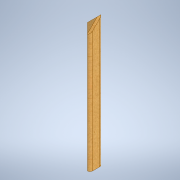
# Autodesk Inventor part: eckeHochkant
Saved by Autodesk Inventor 2020 (Build 240168000, 168)
## iProperties
Created: 2022-03-26
Part Number: eckeHochkant
Material: Kiefer
Document SubType Name: Modeling
Designer: Eric
Density: 0.570257 g/cm^3
Appearance: Gelbkiefer - massiv - natur - schwacher Glanz
Author: Eric
Autodesk Inventor part; units mm, degrees
ref_plane "YZ Plane" through (0, 0, 0) normal (1, 0, 0) x (0, 1, 0)
ref_plane "XZ Plane" through (0, 0, 0) normal (0, 1, 0) x (-1, 0, 0)
ref_plane "XY Plane" through (0, 0, 0) normal (0, 0, 1) x (1, 0, 0)
sketch "Skizze1" plane through (0, 0, 0) normal (0, 1, 0) x (-1, 0, 0)
  arc A0 (-4.6, 0) -> (0, -4.6) centre (0, 0) ccw
  line L0 (-4.6, 0) -> (-4.6, 12.6)
  arc A1 (0, 17.2) -> (-4.6, 12.6) centre (0, 12.6) ccw
  line L1 (0, 17.2) -> (0, 0)
  line L2 (0, 0) -> (17.2, 0)
  arc A2 (12.6, -4.6) -> (17.2, 0) centre (12.6, 0) ccw
  line L3 (12.6, -4.6) -> (0, -4.6)
  dimension "d0" = 4.6
  dimension "d1" = 21.8
  constraints: 8 end point, 6 point on circle, 4 tangent, 3 centre point, 2 equal radius, 2 parallel, 2 perpendicular, 1 coincident, 1 line through centre, 1 point on line, 1 vertical
  measures "d0" distance between parallel lines of L1 L0
  measures "d1" distance from line of L2.end L0
extrude "Extrusion1" add sketch "Skizze1" along normal blind 248.6
sketch "Skizze2" plane through (4.6, 0, 12.6) normal (1, 0, 0) x (0, 0, -1)
  line L0 (17.2, 0) -> (17.2, 248.6) projected
  line L1 (17.2, 248.6) -> (-4.6, 226.8)
  line L2 (-4.6, 0) -> (-4.6, 248.6) projected
  line L3 (-4.6, 226.8) -> (-4.6, 248.6)
  line L4 (17.2, 248.6) -> (12.6, 248.6) projected
  line L5 (-4.6, 248.6) -> (17.2, 248.6)
  point P0 (12.6, 0)
  dimension "d4" = 45
  constraints: 6 end point, 1 perpendicular, 1 point on line, 1 vertical
  measures "d4" angle of L4 L1
extrude "Extrusion2" cut sketch "Skizze2" against normal through all
sketch "Skizze3" plane through (0, 0, -4.6) normal (0, 0, -1) x (-1, 0, 0)
  line L0 (-4.6, 0) -> (-4.6, 244) projected
  line L1 (17.2, 248.6) -> (-4.6, 248.6)
  line L2 (-4.6, 248.6) -> (17.2, 226.8)
  line L3 (17.2, 0) -> (17.2, 244) projected
  line L4 (17.2, 248.6) -> (17.2, 226.8)
  point P0 (0, 0)
  point P1 (0, 248.6)
  dimension "d9" = 45
  constraints: 6 end point, 1 collinear, 1 horizontal, 1 horizontal alignment, 1 point on line, 1 vertical alignment
  measures "d9" angle of L1 L2
extrude "Extrusion3" cut sketch "Skizze3" against normal through all
